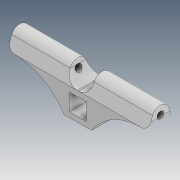
# Autodesk Inventor part: AL_PipeMount
Saved by Autodesk Inventor 2021.4 (Build 254397000, 397)
## iProperties
Created: 2022-02-25
Part Number: AL_PipeMount
Material: Generisch
Document SubType Name: Modeling
Designer: eagle
Density: 1 g/cm^3
Appearance: Vorgabe
Author: eagle
Autodesk Inventor part; units mm, degrees
ref_plane "YZ Plane" through (0, 0, 0) normal (1, 0, 0) x (0, 1, 0)
ref_plane "XZ Plane" through (0, 0, 0) normal (0, 1, 0) x (-1, 0, 0)
ref_plane "XY Plane" through (0, 0, 0) normal (0, 0, 1) x (1, 0, 0)
sketch "Skizze1" plane through (0, 0, 0) normal (0, 0, 1) x (1, 0, 0)
  line L0 (-5.275, 5.275) -> (5.275, 5.275)
  line L1 (5.275, 5.275) -> (5.275, -5.275)
  line L2 (5.275, -5.275) -> (-5.275, -5.275)
  line L3 (-5.275, -5.275) -> (-5.275, 5.275)
  line L4 (-5.275, 5.275) -> (5.275, -5.275) construction
  line L5 (5.275, 5.275) -> (-5.275, -5.275) construction
  line L6 (8.475, 8.475) -> (-8.475, 8.475)
  line L7 (-8.475, 8.475) -> (-8.475, -8.475)
  line L8 (-8.475, -8.475) -> (8.475, -8.475)
  line L9 (8.475, -8.475) -> (8.475, 8.475)
  point P0 (0, 0)
  dimension "d0" = 10.55
  dimension "d1" = 10.55
  dimension "d2" = 3.2
  constraints: 20 end point, 4 parallel, 2 midpoint, 2 perpendicular, 1 horizontal, 3 other
  measures "d0" distance of L1.end L2.end
  measures "d1" distance of L0.end L1.end
  measures "d2" distance between parallel lines of L0 L6
extrude "Extrusion1" add sketch "Skizze1" along normal blind 15
sketch "Skizze2" plane through (8.475, -8.475, 0) normal (1, 0, 0) x (0, 0, -1)
  line L0 (0, 0) -> (0, 16.95) projected
  line L1 (0, 16.95) -> (-15, 16.95) projected
  line L2 (-15, 0) -> (-15, 16.95) projected
  line L3 (0, 0) -> (-15, 0) projected
  circle A0 centre (-7.5, 22) radius 2.1
  circle A1 centre (-7.5, 22) radius 5.3
  line L4 (-15, 16.95) -> (-12.3754, 24.0786)
  line L5 (0, 16.95) -> (0, 0) projected
  line L6 (0, 16.95) -> (-2.5924, 24.0014)
  point P0 (0, 8.475)
  dimension "d5" = 4.2
  dimension "d6" = 22
  dimension "d7" = 7.5
  dimension "d8" = 3.2
  constraints: 4 end point, 2 centre point, 2 point on circle
  measures "d5" diameter of A0
  measures "d6" distance from line of L3 A0.centre
  measures "d7" horizontal distance of L0.start A0.centre
  measures "d8" radial gap between concentric circles of A0 A1
extrude "Extrusion2" add sketch "Skizze2" along normal blind 35 and the other way blind 1 contours L6 L1 A1 | L1 A1 L4 | L4 A1 L1
sketch "Skizze3" plane through (-8.475, -8.475, 0) normal (-1, 0, 0) x (0, 0, 1)
  line L0 (15, 16.95) -> (12.3754, 24.0786) projected
  arc A0 (12.3754, 24.0786) -> (2.5924, 24.0014) centre (7.5, 22) ccw projected
  line L1 (2.5924, 24.0014) -> (0, 16.95) projected
  line L2 (15, 16.95) -> (0, 16.95) projected
  circle A1 centre (7.5, 22) radius 2.1 projected
  point P0 (0, 8.475)
extrude "Extrusion3" add sketch "Skizze3" along normal blind 35 and the other way blind 1
fillet "Rundung2" radius 36.25 2 edges at (-8.475, 8.475, 7.5) (8.475, 8.475, 7.5)
fillet "Rundung5" radius 7 2 edges at (7.475, 8.475, 7.5) (-7.475, 8.475, 7.5)
fillet "Rundung6" radius 4.25 2 edges at (43.475, 8.475, 7.5) (-43.475, 8.475, 7.5)
equation "\"d1\" = d0"
